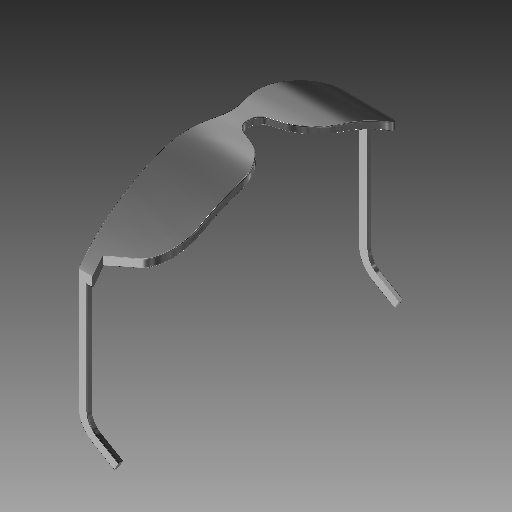
# Autodesk Inventor part: 3D HUMAN
Saved by Autodesk Inventor 2019 (Build 230136000, 136)
## iProperties
Category: PART
Shininess: 64.0
Length Units: 11272
Angle Units: 11279
Time Units: 11290
Mass Units: 11286
Length Display Precision: 3
Angle Display Precision: 2
Compacted: True
Part Number: 3D HUMAN
Document SubType Name: Modeling
Created: 2003-03-24
Designer: M.F.
Catalog Web Link: www.apollocanard.com
Density: 1 g/cm^3
Material: Generic
Appearance: Chrome - Polished Black
Density: 0.0
Volumn: 0.0
Area: 0.0
PropertySet Name: Model Information
Control State: 0
Master: False
Checked Out: False
Title: iMan
Author: M.F.
Autodesk Inventor part; units mm, degrees
ref_plane "YZ Plane" through (0, 0, 0) normal (1, 0, 0) x (0, 1, 0)
ref_plane "XZ Plane" through (0, 0, 0) normal (0, 1, 0) x (-1, 0, 0)
ref_plane "XY Plane" through (0, 0, 0) normal (0, 0, 1) x (1, 0, 0)
sketch "Sketch2" plane through (0, 0, 0) normal (0, 0, 1) x (1, 0, 0)
  line L0 (-59.9849, -29.0944) -> (0, -29.0944)
  line L1 (0, -29.0944) -> (0, 19.3963)
  line L2 (0, 19.3963) -> (-96.9814, 19.3963)
  line L3 (-96.9814, 19.3963) -> (-96.9814, -29.0944)
  line L4 (0, 0) -> (-6.35, 0)
  line L5 (-6.35, 0) -> (-16.9395, -29.0944)
  line L6 (0, 10.5717) -> (-24.2454, 19.3963)
  line L7 (-96.9814, 9.6981) -> (-89.8694, 9.6981)
  line L8 (-89.8694, 9.6981) -> (-84.5194, -10.2684)
  arc A0 (-84.5194, -10.2684) -> (-59.9849, -29.0944) centre (-59.9849, -3.6944) ccw
  point P0 (-79.475, -29.0944)
  dimension "d16" = 20
  dimension "d17" = 6.35
  dimension "d18" = 48.4907
  dimension "d19" = 96.9814
  dimension "d20" = 19.3963
  dimension "d21" = 24.2453
  dimension "d39" = 9.6981
  dimension "d40" = 15
  dimension "d56" = 25.4
  dimension "d57" = 7.112
  constraints: 18 end point, 8 point on line, 3 parallel, 3 perpendicular, 2 point on circle, 2 tangent, 1 centre point, 1 coincident, 1 horizontal
  measures "d16" angle of L1 L5
  measures "d17" distance of L4.start L4.end
  measures "d18" distance of L2.end L3.end
  measures "d19" distance of L1.end L2.end
  measures "d20" distance between parallel lines of L2 L4
  measures "d21" horizontal distance of L6.start L6.end
  measures "d39" distance between parallel lines of L2 L7
  measures "d40" angle of L3 L8
  measures "d56" radius of A0
  measures "d57" distance of L7.start L7.end
extrude "Extrusion1" add sketch "Sketch2" along normal blind 96.9814 contours A0 L8 L7 L3 L2 L6 L1 L4 L5 L0
mirror "Mirror1" about plane through (0, 0, 0) normal (1, 0, 0) of "Extrusion1"
sketch "Sketch3" plane through (-96.9814, 19.3963, 0) normal (0, 1, 0) x (1, 0, 0)
  line L0 (0, 0) -> (0, -96.9814) projected
  line L1 (193.9628, -96.9814) -> (121.2268, -96.9814) projected
  line L2 (193.9628, 0) -> (193.9628, -96.9814) projected
  line L3 (121.2268, 0) -> (193.9628, 0) projected
  line L4 (121.2268, 0) -> (121.2268, -96.9814) projected
  arc A0 (0, 0) -> (193.9628, 0) centre (96.9814, 64.3302) ccw
  arc A1 (0, -8.2615) -> (193.9628, -8.2615) centre (96.9814, 64.3302) ccw
  dimension "d24" = 116.3777
  dimension "d25" = 4.7625
  constraints: 4 point on circle, 2 centre point, 2 point on line
  measures "d24" radius of A0
  measures "d25" radial gap between concentric circles of A1 A0
extrude "Extrusion2" cut sketch "Sketch3" against normal through all contours A0 L4 A1 L0 | A0 L2 A1 L4 keep common part
fillet "Fillet1" radius 7.2736 2 edges at (6.35, 0, 54.2588) (-6.35, 0, 54.2588)
fillet "Fillet1" radius 25.4 3 edges at (-16.9395, -29.0944, 53.2139) (16.9395, -29.0944, 53.2139) (0, 10.5717, 54.4288)
fillet "Fillet1" radius 76.2 2 edges at (-24.2454, 19.3963, 51.9264) (24.2454, 19.3963, 51.9264)
sketch "Sketch4" plane through (-96.9814, 19.3963, 0) normal (-1, 0, 0) x (0, 0, 1)
  line L0 (8.2615, 0) -> (-84.1018, 0)
  line L1 (-84.1018, 0) -> (-84.1018, -6.3038)
  line L2 (-84.1018, -6.3038) -> (8.2615, -6.3038)
  line L3 (8.2615, -6.3038) -> (8.2615, 0)
  line L4 (-84.1018, 0) -> (-98.2798, -24.5571)
  line L5 (-98.2798, -24.5571) -> (-92.8206, -27.709)
  line L6 (-92.8206, -27.709) -> (-80.4623, -6.3038)
  dimension "d29" = 6.3038
  dimension "d30" = 92.3632
  dimension "d31" = 30
  dimension "d37" = 27.709
  constraints: 14 end point, 3 parallel, 2 perpendicular, 1 equal length, 1 horizontal, 1 point on line
  measures "d29" distance of L0.end L1.end
  measures "d30" distance of L0.start L0.end
  measures "d31" angle of L4 L1
  measures "d37" distance from line of L0 L5.end
extrude "Extrusion3" add sketch "Sketch4" against normal blind 3.175
fillet "Fillet2" radius 19.05 1 edges at (-95.3939, 19.3963, -84.1018)
fillet "Fillet2" radius 12.7 1 edges at (-95.3939, 13.0925, -80.4623)
mirror "Mirror2" about plane through (0, 0, 0) normal (1, 0, 0) of "Extrusion3", "Fillet2"
fillet "Fillet3" [suppressed]
fillet "Fillet4" radius 0.7937 39 edges at (-96.9814, 19.3963, -32.4209) (70.611, 19.3963, 34.1027) (-70.611, 19.3963, 34.1027) (-68.9004, 19.3963, 29.4595) (68.9004, 19.3963, 29.4595) (-93.8064, 19.3963, -34.2779) (-96.9814, 16.8441, -82.6282) (-96.9814, 2.3552, -93.9404) (-10.1542, 14.2675, 56.3837) (10.1542, 14.2675, 56.3837) (-10.1542, 14.2675, 51.6037) (10.1542, 14.2675, 51.6037) (93.8064, 19.3963, -34.2779) (93.8064, 16.8441, -82.6282) (93.8064, 2.3552, -93.9404) (-93.8064, 16.8441, -82.6282) (-93.8064, 2.3552, -93.9404) (96.9814, 16.8441, -82.6282) (96.9814, 19.3963, -32.4209) (96.9814, 14.5472, 8.2615) (96.9814, 11.3953, 0) (96.9814, 13.0925, -36.565) (96.9814, -0.7851, -88.4745) (96.9814, -6.7367, -95.5502) (96.9814, 2.3552, -93.9404) (47.6623, -29.0944, 47.0397) (9.4749, -8.5855, 56.4389) (0, 0, 56.81) (-9.4749, -8.5855, 56.4389) (-47.6623, -29.0944, 47.0397) (-96.9814, 14.5472, 8.2615) (47.6936, -29.0944, 41.8258) (9.4749, -8.5857, 51.6612) (0, 0, 52.0475) (-9.4749, -8.5857, 51.6612) (-47.6936, -29.0944, 41.8258) (-96.9814, 11.3953, 0) (-96.9814, 13.0925, -36.565) (-96.9814, -0.7851, -88.4745)
equation "\"d18\" = 0.5 * d19"
equation "\"d20\" = 0.2 * d19"
equation "\"d39\" = 0.2 * d18"
equation "\"d22\" = d19"
equation "\"d24\" = 0.6 * HEAD_TOP_WD"
equation "\"d29\" = 0.065 * d19"
equation "\"d37\" = 0.3 * d30"
equation "\"HEAD_TOP_WD\" = 193.962833"
body "Solid1"
